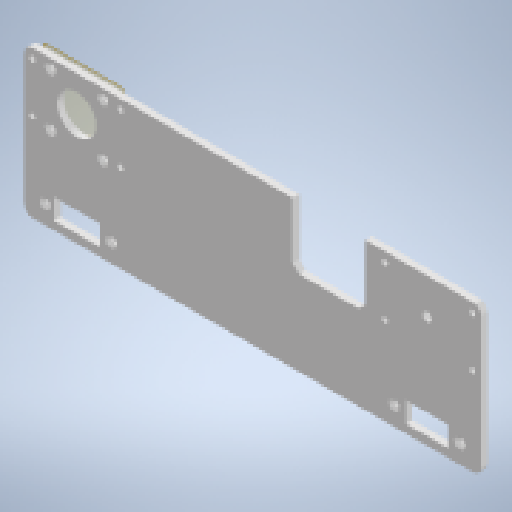
# Autodesk Inventor part: plate_1
Saved by Autodesk Inventor 2024 (Build 280153000, 153)
## iProperties
Created: 2026-02-04
Part Number: plate_1
Material: Generic
Document SubType Name: Modeling
Designer: SEMEN
Density: 1 g/cm^3
Appearance: Default
Author: SEMEN
Autodesk Inventor part; units mm, degrees
ref_plane "YZ Plane" through (0, 0, 0) normal (1, 0, 0) x (0, 1, 0)
ref_plane "XZ Plane" through (0, 0, 0) normal (0, 1, 0) x (-1, 0, 0)
ref_plane "XY Plane" through (0, 0, 0) normal (0, 0, 1) x (1, 0, 0)
ref_plane "Work Plane1" through (0, 0, 0) normal (0, 0, 1) x (1, 0, 0)
sketch "Sketch1" plane through (0, 0, 0) normal (0, 0, 1) x (1, 0, 0)
  circle A0 centre (15.5, -15.5) radius 1.7 projected
  circle A1 centre (15.5, 15.5) radius 1.7 projected
  circle A2 centre (-15.5, 15.5) radius 1.7 projected
  circle A3 centre (-15.5, -15.5) radius 1.7 projected
  circle A4 centre (0, 0) radius 11 projected
  line L0 (17.5, 21) -> (21, 17.5) projected
  line L1 (17.5, 21) -> (-17.5, 21) projected
  line L2 (-21, 17.5) -> (-17.5, 21) projected
  line L3 (-21, 17.5) -> (-21, -17.5) projected
  line L4 (-17.5, -21) -> (-21, -17.5) projected
  line L5 (-17.5, -21) -> (17.5, -21) projected
  line L6 (21, -17.5) -> (17.5, -21) projected
  line L7 (21, -17.5) -> (21, 17.5) projected
  line L8 (-31, 21) -> (239, 21)
  line L9 (239, 21) -> (239, -66)
  line L10 (239, -66) -> (-31, -66)
  line L11 (-31, -66) -> (-31, 21)
  circle A5 centre (207, 0) radius 22 construction
  line L12 (0, 0) -> (239, 0) construction
  circle A6 centre (0, 0) radius 11.5
  line L13 (104, 21) -> (104, -66) construction
  line L14 (-15.5, 15.5) -> (-31, 15.5) construction
  line L15 (207, 0) -> (207, -66) construction
  line L16 (0, 0) -> (0, -66) construction
  line L17 (219.5, -49) -> (194.5, -49)
  line L18 (194.5, -49) -> (194.5, -61)
  line L19 (194.5, -61) -> (219.5, -61)
  line L20 (219.5, -61) -> (219.5, -49)
  line L21 (219.5, -49) -> (194.5, -61) construction
  line L22 (194.5, -49) -> (219.5, -61) construction
  line L23 (219.5, -55) -> (194.5, -55) construction
  line L24 (-13.5, -61) -> (13.5, -61)
  line L25 (13.5, -61) -> (13.5, -49)
  line L26 (13.5, -49) -> (-13.5, -49)
  line L27 (-13.5, -49) -> (-13.5, -61)
  line L28 (-13.5, -61) -> (13.5, -49) construction
  line L29 (13.5, -61) -> (-13.5, -49) construction
  line L30 (170, 23) -> (166.5, 26.5) projected
  line L31 (170, 23) -> (170, -12) projected
  line L32 (166.5, -15.5) -> (170, -12) projected
  line L33 (166.5, -15.5) -> (131.5, -15.5) projected
  line L34 (128, -12) -> (131.5, -15.5) projected
  line L35 (128, -12) -> (128, 23) projected
  line L36 (131.5, 26.5) -> (128, 23) projected
  line L37 (131.5, 26.5) -> (166.5, 26.5) projected
  line L38 (127.5, 23.2071) -> (127.5, -12.2071)
  line L39 (127.5, -12.2071) -> (131.2929, -16)
  line L40 (131.2929, -16) -> (166.7071, -16)
  line L41 (166.7071, -16) -> (170.5, -12.2071)
  line L42 (170.5, -12.2071) -> (170.5, 23.2071)
  line L43 (170.5, 23.2071) -> (166.7071, 27)
  line L44 (166.7071, 27) -> (131.2929, 27)
  line L45 (131.2929, 27) -> (127.5, 23.2071)
  line L46 (-32.0916, -17) -> (139.8961, -17) construction
  point P0 (-26, 15.5)
  point P1 (-26, -14)
  point P2 (234, 15.5)
  point P3 (234, -14)
  point P4 (207, -55)
  point P5 (226.5, -55)
  point P6 (187.5, -55)
  point P7 (0, -55)
  point P8 (20.5, -55)
  point P9 (-18.5, -55)
  point P10 (26, 15.5)
  point P11 (26, -14)
  point P12 (182, 15.5)
  point P13 (182, -14)
  point P14 (170.5, 21)
  point P15 (127.5, 21)
  dimension "d0" = 45
  dimension "d1" = 270
  dimension "d2" = 44
  dimension "d3" = 0.5
  dimension "d21" = 10
  dimension "d22" = 32
  dimension "d23" = 5
  dimension "d31" = 25
  dimension "d32" = 12
  dimension "d33" = 5
  dimension "d34" = 7
  dimension "d42" = 0.5
  dimension "d50" = 5
  dimension "d51" = 17
  dimension "d52" = 3
  constraints: 62 end point, 9 point on line, 9 symmetric about line, 8 midpoint, 6 parallel, 6 perpendicular, 4 horizontal, 3 collinear, 2 centre point, 1 vertical, 8 other
  measures "d0" distance between parallel lines of L10 L5
  measures "d1" distance between parallel lines of L9 L11
  measures "d2" diameter of A5
  measures "d3" radial gap between concentric circles of A4 A6
  measures "d21" distance between parallel lines of L11 L3
  measures "d22" distance from line of L9 L15.start
  measures "d23" distance from line of L11 point (-26, 15.5)
  measures "d31" distance of L19.end L18.end
  measures "d32" distance of L18.end L17.end
  measures "d33" distance between parallel lines of L10 L19
  measures "d34" distance from line of L20 point (226.5, -55)
  measures "d42" distance between parallel lines of L35 L38
  measures "d50" distance from line of L11 point (-26, -14)
  measures "d51" distance from line of L46 point (0, 0)
  measures "d52" distance from line of L46 point (-26, -14)
extrude "Extrusion1" add sketch "Sketch1" along normal blind 4 contours A0 | A1 | A2 | A3 | L8 L38 L39 L40 L41 L42 L9 L10 L11 L2 L3 L4 L5 L6 L7 L0 | L0 L7 L6 L5 L4 L3 L2 L1
hole "Hole1" at (207, 0, 0) direction (0, 0, 1) diameter 5.5 end through all clearance for "Countersunk Head GOST 12876-67" size "M5" standard "GOST"
sketch "Sketch2" plane through (0, 0, 4) normal (0, 0, 1) x (1, 0, 0)
  circle A0 centre (15.5, -15.5) radius 1.7 projected
  circle A1 centre (15.5, 15.5) radius 1.7 projected
  circle A2 centre (-15.5, 15.5) radius 1.7 projected
  circle A3 centre (-15.5, -15.5) radius 1.7 projected
  circle A4 centre (0, 0) radius 11 projected
  line L0 (17.5, 21) -> (21, 17.5) projected
  line L1 (17.5, 21) -> (-17.5, 21) projected
  line L2 (-21, 17.5) -> (-17.5, 21) projected
  line L3 (-21, 17.5) -> (-21, -17.5) projected
  line L4 (-17.5, -21) -> (-21, -17.5) projected
  line L5 (-17.5, -21) -> (17.5, -21) projected
  line L6 (21, -17.5) -> (17.5, -21) projected
  line L7 (21, -17.5) -> (21, 17.5) projected
  point P0 (-18.5, -55)
  point P1 (20.5, -55)
  point P2 (187.5, -55)
  point P3 (226.5, -55)
hole "Hole2" at (-15.5, -15.5, 4) at (-15.5, 15.5, 4) at (15.5, 15.5, 4) at (15.5, -15.5, 4) direction (0, 0, -1) diameter 3.4 end through all countersink diameter 6.6 countersink angle 90 clearance for "Countersunk Head GOST 12876-67" size "M3" standard "GOST"
fillet "Fillet1" radius 5 4 edges at (-31, 21, 2) (-31, -66, 2) (239, 21, 2) (239, -66, 2)
hole "Hole3" at (-26, -14, 0) at (-26, 15.5, 0) at (234, 15.5, 0) at (234, -14, 0) at (26, 15.5, 0) at (26, -14, 0) direction (0, 0, 1) diameter 3.4 end through all countersink diameter 6.6 countersink angle 90 clearance for "Countersunk Head GOST 12876-67" size "M3" standard "GOST"
hole "Hole4" at (-18.5, -55, 4) at (20.5, -55, 4) at (187.5, -55, 4) at (226.5, -55, 4) direction (0, 0, -1) diameter 3.4 end through all countersink diameter 6.6 countersink angle 90 clearance for "Countersunk Head GOST 12876-67" size "M3" standard "GOST"
hole "Hole5" at (182, 15.5, 0) at (182, -14, 0) direction (0, 0, 1) diameter 3.4 end through all clearance for "Countersunk Head GOST 12876-67" size "M3" standard "GOST"
body "Solid1"
